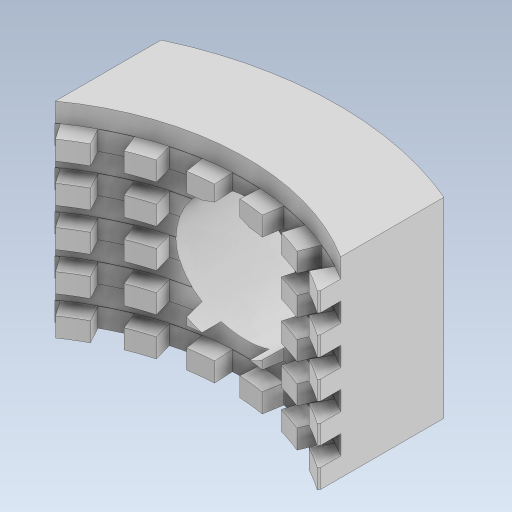
# Autodesk Inventor part: Plunger Cap
Saved by Autodesk Inventor 2023 (Build 270158000, 158)
## iProperties
Created: 2022-09-14
Part Number: Plunger Cap
Material: Generic
Document SubType Name: Modeling
Designer: Dave
Density: 1 g/cm^3
Appearance: Default
Author: Dave
## iProperties of the stored document Plunger Cap_3DPrint.ipt
Created: 2022-09-16
Part Number: Plunger Cap_3DPrint
Material: Generic
Document SubType Name: Modeling
Designer: Dave
Density: 1 g/cm^3
Appearance: Default
Author: Dave
Autodesk Inventor part; units mm, degrees
ref_plane "YZ Plane" through (0, 0, 0) normal (1, 0, 0) x (0, 1, 0)
ref_plane "XZ Plane" through (0, 0, 0) normal (0, 1, 0) x (-1, 0, 0)
sketch "Sketch1" plane through (0, 0, 0) normal (0, 1, 0) x (-1, 0, 0)
  arc A0 (16.222958, 7.3) -> (7.325, 16.197958) centre (0, -0.025) ccw
  line L0 (7.325, 16.197958) -> (7.325, 21.125)
  arc A1 (7.325, 21.125) -> (7.025, 22.178565) centre (5.325, 21.125) ccw
  arc A2 (7.025, 22.178565) -> (6.378565, 22.825) centre (5.325, 21.125) ccw
  arc A3 (6.378565, 22.825) -> (5.325, 23.125) centre (5.325, 21.125) ccw
  line L1 (5.325, 23.125) -> (-5.325, 23.125)
  arc A4 (-5.325, 23.125) -> (-6.378565, 22.825) centre (-5.325, 21.125) ccw
  arc A5 (-6.378565, 22.825) -> (-7.025, 22.178565) centre (-5.325, 21.125) ccw
  arc A6 (-7.025, 22.178565) -> (-7.325, 21.125) centre (-5.325, 21.125) ccw
  line L2 (-7.325, 21.125) -> (-7.325, 16.197958)
  arc A7 (-7.325, 16.197958) -> (-16.222958, 7.3) centre (0, -0.025) ccw
  line L3 (-16.222958, 7.3) -> (-21.147255, 7.3)
  ellipse E0 centre (-21.252071, 5.3) end of major axis (-19.761801, 6.714214) minor radius 1.949633 (-21.147255, 7.3) -> (-22.217989, 7) ccw
  ellipse E1 centre (-21.162978, 5.3) end of major axis (-23.165722, 5.3) minor radius 2 (-22.217989, 7) -> (-22.85, 6.377846) ccw
  ellipse E2 centre (-21.246988, 5.3) end of major axis (-21.246988, 7.3) minor radius 1.903012 (-22.85, 6.377846) -> (-23.15, 5.3) ccw
  line L4 (-23.15, 5.3) -> (-23.15, -5.35)
  ellipse E3 centre (-21.246988, -5.35) end of major axis (-21.246988, -3.35) minor radius 1.903012 (-23.15, -5.35) -> (-22.85, -6.427846) ccw
  ellipse E4 centre (-21.162978, -5.35) end of major axis (-23.165722, -5.35) minor radius 2 (-22.85, -6.427846) -> (-22.217989, -7.05) ccw
  ellipse E5 centre (-21.252071, -5.35) end of major axis (-22.742341, -3.935786) minor radius 1.949633 (-22.217989, -7.05) -> (-21.147255, -7.35) ccw
  line L5 (-21.147255, -7.35) -> (-16.222958, -7.35)
  arc A8 (-16.222958, -7.35) -> (-7.325, -16.247958) centre (0, -0.025) ccw
  line L6 (-7.325, -16.247958) -> (-7.325, -21.175)
  line L7 (-7.025, -22.228565) -> (-7.025, -16.053081)
  arc A9 (-7.325, -21.175) -> (-7.025, -22.228565) centre (-5.325, -21.175) ccw
  arc A10 (-7.025, -22.228565) -> (-6.378565, -22.875) centre (-5.325, -21.175) ccw
  arc A11 (-6.378565, -22.875) -> (-5.325, -23.175) centre (-5.325, -21.175) ccw
  line L8 (-5.325, -23.175) -> (5.325, -23.175)
  line L9 (7.325, -21.175) -> (7.325, -16.247958)
  arc A12 (7.025, -22.228565) -> (7.325, -21.175) centre (5.325, -21.175) ccw
  arc A13 (6.378565, -22.875) -> (7.025, -22.228565) centre (5.325, -21.175) ccw
  arc A14 (5.325, -23.175) -> (6.378565, -22.875) centre (5.325, -21.175) ccw
  arc A15 (7.325, -16.247958) -> (16.222958, -7.35) centre (0, -0.025) ccw
  line L10 (16.222958, -7.35) -> (21.147255, -7.35)
  ellipse E6 centre (21.252071, -5.35) end of major axis (19.761801, -6.764214) minor radius 1.949633 (21.147255, -7.35) -> (22.217989, -7.05) ccw
  ellipse E7 centre (21.162978, -5.35) end of major axis (23.165722, -5.35) minor radius 2 (22.217989, -7.05) -> (22.85, -6.427846) ccw
  ellipse E8 centre (21.246988, -5.35) end of major axis (21.246988, -7.35) minor radius 1.903012 (22.85, -6.427846) -> (23.15, -5.35) ccw
  line L11 (23.15, -5.35) -> (23.15, 5.3)
  ellipse E9 centre (21.246988, 5.3) end of major axis (21.246988, 3.3) minor radius 1.903012 (23.15, 5.3) -> (22.85, 6.377846) ccw
  ellipse E10 centre (21.162978, 5.3) end of major axis (23.165722, 5.3) minor radius 2 (22.85, 6.377846) -> (22.217989, 7) ccw
  ellipse E11 centre (21.252071, 5.3) end of major axis (22.742341, 3.885786) minor radius 1.949633 (22.217989, 7) -> (21.147255, 7.3) ccw
  line L12 (21.147255, 7.3) -> (16.222958, 7.3)
  circle A16 centre (0, -0.025) radius 13
  point P0 (0, 0)
  point P1 (0, 0)
  dimension "d0" = 26
  constraints: 32 point on circle, 26 end point, 17 centre point, 1 coincident, 1 vertical, 49 other
  measures "d0" diameter of A16
extrude "Extrusion1" add sketch "Sketch1" along normal blind 6
sketch "Sketch2" plane through (0, 6, 0) normal (0, 1, 0) x (1, 0, 0)
  circle A0 centre (0, 0.025) radius 13
  line L0 (-13, 0.025) -> (-17.8, 0.025)
  arc A1 (17.8, 0.025) -> (-17.8, 0.025) centre (0, 0.025) ccw
  arc A2 (-7.325, 16.247958) -> (-16.222958, 7.35) centre (0, 0.025) ccw
  line L1 (13, 0.025) -> (17.8, 0.025)
  line L2 (-15.415252, 8.925) -> (-10.392305, 6.025)
  line L3 (10.392305, 6.025) -> (15.415252, 8.925)
  arc A3 (16.222958, 7.35) -> (7.325, 16.247958) centre (0, 0.025) ccw
  line L4 (0, 32.435) -> (0, -32.385)
  circle A4 centre (0, 0.025) radius 12
  point P0 (0, 0)
  point P1 (-11.25833, 6.525)
  point P2 (11.25833, 6.525)
  dimension "d3" = 120
  dimension "d6" = 1
  constraints: 10 point on circle, 8 end point, 2 centre point, 2 coincident, 2 horizontal, 2 horizontal alignment, 2 point on line, 1 concentric, 1 line through centre, 1 other
  measures "d3" angle of L3 L2
  measures "d6" radial gap between concentric circles of A0 A4
extrude "Extrusion2" add sketch "Sketch2" along normal blind 10 contours L3 A4 L4 A0 | A0 L4 A1 L3 | L4 A4 L2 A0 | A0 L2 A1 L4 picked at (0.900951, 12.596973) picked at (-0.900951, 12.596973)
sketch "Sketch3" plane through (0, 16, 0) normal (0, 1, 0) x (1, 0, 0)
  arc A0 (10.392305, 6.025) -> (-10.392305, 6.025) centre (0, 0.025) ccw
  circle A1 centre (0, 0) radius 12.01252
  line L0 (-11.25833, 6.525) -> (-10.392305, 6.025)
  circle A2 centre (0, 0) radius 13.012518
  line L1 (-10.392305, 6.025) -> (-11.25833, 6.525)
  arc A3 (11.25833, 6.525) -> (-11.25833, 6.525) centre (0, 0.025) ccw
  line L2 (-9.666431, 7.131671) -> (-10.472196, 7.723907)
  line L3 (-8.82322, 8.151774) -> (-9.558944, 8.829055)
  line L4 (-7.872907, 9.072925) -> (-8.529659, 9.827031)
  line L5 (-6.827027, 9.883943) -> (-7.396835, 10.705721)
  line L6 (-5.698277, 10.574983) -> (-6.174224, 11.454457)
  line L7 (-4.500357, 11.137657) -> (-4.876667, 12.064151)
  line L8 (-3.247809, 11.565136) -> (-3.519913, 12.527404)
  line L9 (-1.955837, 11.852229) -> (-2.120432, 12.83859)
  line L10 (-0.640124, 11.995452) -> (-0.695212, 12.993933)
  line L11 (0.683359, 11.993067) -> (0.738447, 12.991548)
  line L12 (1.998548, 11.845102) -> (2.163142, 12.831463)
  line L13 (3.289477, 11.553353) -> (3.56158, 12.515621)
  line L14 (4.540476, 11.121363) -> (4.916785, 12.047857)
  line L15 (5.736359, 10.554374) -> (6.212307, 11.433848)
  line L16 (6.862611, 9.859269) -> (7.432419, 10.681047)
  line L17 (7.905561, 9.044487) -> (8.562313, 9.798593)
  line L18 (8.852547, 8.119916) -> (9.588271, 8.797198)
  line L19 (9.692076, 7.096781) -> (10.497841, 7.689016)
  line L20 (10.413955, 5.9875) -> (11.279981, 6.4875)
  point P0 (0.00275, 0.024848)
  point P1 (0.005467, 0.024395)
  point P2 (0.008117, 0.023645)
  point P3 (0.010669, 0.022609)
  point P4 (0.013092, 0.021298)
  point P5 (0.015355, 0.019729)
  point P6 (0.017432, 0.01792)
  point P7 (0.019298, 0.015893)
  point P8 (0.020929, 0.013674)
  point P9 (0.022306, 0.011288)
  point P10 (0.023413, 0.008766)
  point P11 (0.024235, 0.006137)
  point P12 (0.024763, 0.003434)
  point P13 (0.024991, 0.000689)
  point P14 (0.024915, -0.002064)
  point P15 (0.024536, -0.004793)
  point P16 (0.02386, -0.007463)
  point P17 (0.022894, -0.010042)
  point P18 (0.021651, -0.0125)
  point P19 (9.693875, 7.098103)
  point P20 (8.855759, 8.122872)
  point P21 (7.909693, 9.049232)
  point P22 (6.867165, 9.865836)
  point P23 (5.740852, 10.562676)
  point P24 (4.544473, 11.131204)
  point P25 (3.292612, 11.564441)
  point P26 (2.000545, 11.857067)
  point P27 (0.684045, 12.005488)
  point P28 (-0.64081, 12.007878)
  point P29 (-1.957836, 11.864209)
  point P30 (-3.250951, 11.576247)
  point P31 (-4.504367, 11.14753)
  point P32 (-5.70279, 10.583323)
  point P33 (-6.83161, 9.890552)
  point P34 (-7.877078, 9.077714)
  point P35 (-8.82648, 8.154775)
  point P36 (-9.668289, 7.133037)
  dimension "d9" = 120
  constraints: 40 end point, 3 point on circle, 2 coincident, 1 centre point, 80 other
sketch "Sketch3 outline for Extrusion3" plane through (0, 16, 0) normal (0, 1, 0) x (1, 0, 0)
  line L0 (9.693875, 7.098103) -> (10.497841, 7.689016)
  arc A0 (8.855759, 8.122872) -> (9.693875, 7.098103) centre (0, 0.025) cw
  line L1 (9.588271, 8.797198) -> (8.855759, 8.122872)
  arc A1 (10.497841, 7.689016) -> (9.588271, 8.797198) centre (0, 0) ccw
  line L2 (7.909693, 9.049232) -> (8.562313, 9.798593)
  arc A2 (6.867165, 9.865836) -> (7.909693, 9.049232) centre (0, 0.025) cw
  line L3 (7.432419, 10.681047) -> (6.867165, 9.865836)
  arc A3 (8.562313, 9.798593) -> (7.432419, 10.681047) centre (0, 0) ccw
  line L4 (5.740852, 10.562676) -> (6.212307, 11.433848)
  arc A4 (4.544473, 11.131204) -> (5.740852, 10.562676) centre (0, 0.025) cw
  line L5 (4.916785, 12.047857) -> (4.544473, 11.131204)
  arc A5 (6.212307, 11.433848) -> (4.916785, 12.047857) centre (0, 0) ccw
  line L6 (3.292612, 11.564441) -> (3.56158, 12.515621)
  arc A6 (2.000545, 11.857067) -> (3.292612, 11.564441) centre (0, 0.025) cw
  line L7 (2.163142, 12.831463) -> (2.000545, 11.857067)
  arc A7 (3.56158, 12.515621) -> (2.163142, 12.831463) centre (0, 0) ccw
  line L8 (0.684045, 12.005488) -> (0.738447, 12.991548)
  arc A8 (-0.64081, 12.007878) -> (0.684045, 12.005488) centre (0, 0.025) cw
  line L9 (-0.695212, 12.993933) -> (-0.64081, 12.007878)
  arc A9 (0.738447, 12.991548) -> (-0.695212, 12.993933) centre (0, 0) ccw
  line L10 (-1.957836, 11.864209) -> (-2.120432, 12.83859)
  arc A10 (-3.250951, 11.576247) -> (-1.957836, 11.864209) centre (0, 0.025) cw
  line L11 (-3.519913, 12.527404) -> (-3.250951, 11.576247)
  arc A11 (-2.120432, 12.83859) -> (-3.519913, 12.527404) centre (0, 0) ccw
  line L12 (-4.504367, 11.14753) -> (-4.876667, 12.064151)
  arc A12 (-5.70279, 10.583323) -> (-4.504367, 11.14753) centre (0, 0.025) cw
  line L13 (-6.174224, 11.454457) -> (-5.70279, 10.583323)
  arc A13 (-4.876667, 12.064151) -> (-6.174224, 11.454457) centre (0, 0) ccw
  line L14 (-6.83161, 9.890552) -> (-7.396835, 10.705721)
  arc A14 (-7.877078, 9.077714) -> (-6.83161, 9.890552) centre (0, 0.025) cw
  line L15 (-8.529659, 9.827031) -> (-7.877078, 9.077714)
  arc A15 (-7.396835, 10.705721) -> (-8.529659, 9.827031) centre (0, 0) ccw
  line L16 (-8.82648, 8.154775) -> (-9.558944, 8.829055)
  arc A16 (-9.668289, 7.133037) -> (-8.82648, 8.154775) centre (0, 0.025) cw
  line L17 (-10.472196, 7.723907) -> (-9.668289, 7.133037)
  arc A17 (-9.558944, 8.829055) -> (-10.472196, 7.723907) centre (0, 0) ccw
extrude "Extrusion3" cut sketch "Sketch3 outline for Extrusion3" against normal blind 10
sketch "Sketch4" plane through (15.415252, 6, -8.925) normal (0.5, 0, 0.8660254) x (0.8660254, 0, -0.5)
  line L0 (-5.8, 10) -> (0, 10)
  line L1 (-5.8, 10) -> (-4.8, 10)
  line L2 (-5.8, 0) -> (-4.8, 0)
  line L3 (-5.8, 10) -> (-5.8, 0)
  line L4 (-5.8, 0) -> (-4.8, 0)
  line L5 (-5.498023, 10) -> (-5.498023, 0)
  line L6 (-4.8, 0) -> (-4.8, 10)
  line L7 (-5.8, 9) -> (-4.8, 9)
  line L8 (-5.8, 8) -> (-4.8, 8)
  line L9 (-5.8, 7) -> (-4.8, 7)
  line L10 (-5.8, 6) -> (-4.8, 6)
  line L11 (-5.8, 5) -> (-4.8, 5)
  line L12 (-5.8, 4) -> (-4.8, 4)
  line L13 (-5.8, 3) -> (-4.8, 3)
  line L14 (-5.8, 2) -> (-4.8, 2)
  line L15 (-5.8, 1) -> (-4.8, 1)
  line L16 (-17.8125, -9.2) -> (-17.8125, 13.2)
  line L17 (-7.530511, 10) -> (-6.715561, 10)
  line L18 (-5.8, 0) -> (-6.785248, 0)
  line L19 (-6.785248, 0) -> (-6.785248, 10)
  line L20 (-6.785248, 10) -> (-5.8, 10)
  line L21 (-5.8, 10) -> (-5.8, 0)
  point P0 (-17.8125, -6)
  point P1 (-4.8, 1)
  point P2 (-4.8, 2)
  point P3 (-5.8, 2)
  point P4 (-5.8, 1)
  point P5 (-4.8, 3)
  point P6 (-4.8, 4)
  point P7 (-5.8, 4)
  point P8 (-5.8, 3)
  point P9 (-4.8, 5)
  point P10 (-4.8, 6)
  point P11 (-5.8, 6)
  point P12 (-5.8, 5)
  point P13 (-4.8, 7)
  point P14 (-4.8, 8)
  point P15 (-5.8, 8)
  point P16 (-5.8, 7)
  point P17 (-4.8, 9)
  point P18 (-4.8, 10)
  point P19 (-5.8, 9)
  dimension "d16" = 1
  constraints: 34 end point, 3 equal length, 3 vertical, 2 horizontal, 1 perpendicular, 1 point on line, 27 other
  measures "d16" distance of L0.start L7.start
revolve "Revolution1" cut sketch "Sketch4" angle 360 about axis through (-0.010825, -10, -0.01875) along (0, -1, 0) contours L0 L5 L7 L3 | L3 L18 L19 L17 L20 | L0 L6 L7 L5 | L8 L5 L9 L3 | L8 L6 L9 L5 | L10 L5 L11 L3 | L10 L6 L11 L5 | L3 L14 L5 L15 | L12 L5 L13 L3 | L5 L14 L6 L15 | L12 L6 L13 L5
sketch "Sketch25" plane through (0, 0, 0) normal (0, -1, 0) x (1, 0, 0)
  line L0 (5.325, -23.175) -> (-5.325, -23.175)
  arc A0 (5.325, -23.175) -> (7.325, -21.175) centre (5.325, -21.175) ccw
  line L1 (7.325, -16.247958) -> (7.325, -21.175)
  arc A1 (7.325, -16.247958) -> (16.222958, -7.35) centre (0, -0.025) ccw
  line L2 (21.147255, -7.35) -> (16.222958, -7.35)
  ellipse E0 centre (21.252071, -5.35) end of major axis (22.742341, -3.935786) minor radius 1.949633 (21.147255, -7.35) -> (22.217989, -7.05) ccw
  ellipse E1 centre (21.162978, -5.35) end of major axis (23.165722, -5.35) minor radius 2 (22.217989, -7.05) -> (22.85, -6.427846) ccw
  ellipse E2 centre (21.246988, -5.35) end of major axis (21.246988, -3.35) minor radius 1.903012 (22.85, -6.427846) -> (23.15, -5.35) ccw
  line L3 (23.15, 5.3) -> (23.15, -5.35)
  ellipse E3 centre (21.246988, 5.3) end of major axis (21.246988, 7.3) minor radius 1.903012 (23.15, 5.3) -> (22.85, 6.377846) ccw
  ellipse E4 centre (21.162978, 5.3) end of major axis (23.165722, 5.3) minor radius 2 (22.85, 6.377846) -> (22.217989, 7) ccw
  ellipse E5 centre (21.252071, 5.3) end of major axis (19.761801, 6.714214) minor radius 1.949633 (22.217989, 7) -> (21.147255, 7.3) ccw
  line L4 (16.222958, 7.3) -> (21.147255, 7.3)
  arc A2 (16.222958, 7.3) -> (7.325, 16.197958) centre (0, -0.025) ccw
  line L5 (7.325, 21.125) -> (7.325, 16.197958)
  arc A3 (7.325, 21.125) -> (5.325, 23.125) centre (5.325, 21.125) ccw
  line L6 (-5.325, 23.125) -> (5.325, 23.125)
  arc A4 (-5.325, 23.125) -> (-7.325, 21.125) centre (-5.325, 21.125) ccw
  line L7 (-7.325, 16.197958) -> (-7.325, 21.125)
  arc A5 (-7.325, 16.197958) -> (-16.222958, 7.3) centre (0, -0.025) ccw
  line L8 (-21.147255, 7.3) -> (-16.222958, 7.3)
  ellipse E6 centre (-21.252071, 5.3) end of major axis (-22.742341, 3.885786) minor radius 1.949633 (-21.147255, 7.3) -> (-22.217989, 7) ccw
  ellipse E7 centre (-21.162978, 5.3) end of major axis (-23.165722, 5.3) minor radius 2 (-22.217989, 7) -> (-22.85, 6.377846) ccw
  ellipse E8 centre (-21.246988, 5.3) end of major axis (-21.246988, 3.3) minor radius 1.903012 (-22.85, 6.377846) -> (-23.15, 5.3) ccw
  line L9 (-23.15, -5.35) -> (-23.15, 5.3)
  ellipse E9 centre (-21.246988, -5.35) end of major axis (-21.246988, -7.35) minor radius 1.903012 (-23.15, -5.35) -> (-22.85, -6.427846) ccw
  ellipse E10 centre (-21.162978, -5.35) end of major axis (-23.165722, -5.35) minor radius 2 (-22.85, -6.427846) -> (-22.217989, -7.05) ccw
  ellipse E11 centre (-21.252071, -5.35) end of major axis (-19.761801, -6.764214) minor radius 1.949633 (-22.217989, -7.05) -> (-21.147255, -7.35) ccw
  line L10 (-16.222958, -7.35) -> (-21.147255, -7.35)
  arc A6 (-16.222958, -7.35) -> (-7.325, -16.247958) centre (0, -0.025) ccw
  line L11 (-7.325, -21.175) -> (-7.325, -16.247958)
  arc A7 (-7.325, -21.175) -> (-5.325, -23.175) centre (-5.325, -21.175) ccw
  circle A8 centre (0, -0.025) radius 13
  point P0 (0, 0)
  constraints: 12 other
extrude "Extrusion13" cut sketch "Sketch25" against normal blind 6
ref_plane "Work Plane5" through (11.25833, 15.5, -6.525) normal (0.000416, 0, -0.9999999) x (0, -1, 0)
sketch "Sketch26" plane through (11.25833, 15.5, -6.525) normal (0.000416, 0, -0.9999999) x (0, -1, 0)
  line L0 (9.5, 26.674578) -> (-0.5, 26.674578)
  line L1 (-0.5, 0) -> (-0.5, 22.532897)
  circle A0 centre (4.5, 11.266448) radius 3.25
  point P0 (15.5, 11.255615)
  point P1 (-0.5, 11.266448)
  point P2 (4.5, 26.674578)
  dimension "d107" = 6.5
  constraints: 2 midpoint, 1 centre point, 1 horizontal alignment, 1 vertical alignment
  measures "d107" diameter of A0
extrude "Extrusion14" cut sketch "Sketch26" along normal through all
sketch "Sketch27" plane through (0, 16, 0) normal (0, 1, 0) x (1, 0, 0)
  line L0 (6.939286, 20.258571) -> (-7.560714, 20.258571)
  line L1 (-7.560714, 20.258571) -> (-7.560714, 0)
  line L2 (-7.560714, 0) -> (6.939286, 0)
  line L3 (6.939286, 0) -> (6.939286, 20.258571)
  line L4 (20.340586, 29.241651) -> (-23.901012, 29.241651)
  line L5 (-23.901012, 29.241651) -> (-23.901012, -10.912048)
  line L6 (-23.901012, -10.912048) -> (20.340586, -10.912048)
  line L7 (20.340586, -10.912048) -> (20.340586, 29.241651)
  point P0 (0, 0)
  point P1 (-0.310714, 0)
  dimension "d110" = 14.5
  constraints: 16 end point, 4 parallel, 2 horizontal, 2 perpendicular, 1 horizontal alignment, 1 midpoint
  measures "d110" distance of L1.end L2.end
extrude "Extrusion15" cut sketch "Sketch27" against normal through all
body "Solid1"
